przegub 1 front cover v20 (Autodesk Fusion 360 design; units mm, degrees)
Autodesk Fusion 360 part; units mm, degrees
derive "derive" from "Robot asembly v98"
sketch "Sketch1" plane through (0, -130, 0) normal (0, -1, 0) x (1, 0, 0)
  line L0 (-73, -52.5227) -> (-73, -58.5227)
  line L1 (-73, -58.5227) -> (73, -58.5227)
  line L2 (73, -58.5227) -> (73, -52.5227)
  line L3 (73, -52.5227) -> (68, -52.5227)
  line L4 (-68, -54.5227) -> (-68, -52.5227)
  line L5 (-68, -52.5227) -> (-73, -52.5227)
  line L6 (76, -4.5227) -> (73, -4.5227)
  line L7 (73, -4.5227) -> (73, -58.5227)
  line L8 (73, -58.5227) -> (76, -58.5227)
  line L9 (76, -58.5227) -> (76, -4.5227)
  line L10 (73, -4.5227) -> (76, -4.5227)
  arc A0 (76, -4.5227) -> (70, 1.4773) centre (70, -4.5227) ccw
  line L11 (70, 1.4773) -> (70, -1.5227)
  arc A1 (73, -4.5227) -> (70, -1.5227) centre (70, -4.5227) ccw
  line L12 (70, 1.4773) -> (-70, 1.4773)
  line L13 (-70, 1.4773) -> (-70, -1.5227)
  line L14 (-70, -1.5227) -> (70, -1.5227)
  line L15 (70, -1.5227) -> (70, 1.4773)
  line L16 (-76, -4.5227) -> (-73, -4.5227)
  arc A2 (-70, -1.5227) -> (-73, -4.5227) centre (-70, -4.5227) ccw
  line L17 (-70, -1.5227) -> (-70, 1.4773)
  arc A3 (-70, 1.4773) -> (-76, -4.5227) centre (-70, -4.5227) ccw
  line L18 (-73, -4.5227) -> (-76, -4.5227)
  line L19 (-76, -4.5227) -> (-76, -58.5227)
  line L20 (-76, -58.5227) -> (-73, -58.5227)
  line L21 (-73, -58.5227) -> (-73, -4.5227)
  line L22 (69, -5.5227) -> (69, -59.157)
  line L23 (-69, -5.5227) -> (69, -5.5227)
  line L24 (-69, -59.157) -> (-69, -5.5227)
  circle A4 centre (55, -28.5227) radius 12
  line L25 (68.85, -12.1227) -> (41.15, -12.1227) construction
  line L26 (41.15, -12.1227) -> (41.15, -44.9227) construction
  line L27 (41.15, -44.9227) -> (68.85, -44.9227) construction
  line L28 (68.85, -44.9227) -> (68.85, -12.1227) construction
  line L29 (68.85, -12.1227) -> (41.15, -44.9227) construction
  line L30 (41.15, -12.1227) -> (68.85, -44.9227) construction
  circle A5 centre (45.3218, -17.0626) radius 2
  circle A6 centre (64.6782, -39.9828) radius 2
  line L31 (55, -28.5227) -> (68.85, -16.8262) construction
  line L32 (30.15, -12.5227) -> (30.15, -44.5227) construction
  circle A7 centre (30.15, -44.5227) radius 2
  circle A8 centre (30.15, -12.5227) radius 2
  line L33 (24.65, -17.0227) -> (35.65, -17.0227)
  line L34 (24.65, -17.0227) -> (24.65, -40.0227)
  line L35 (24.65, -40.0227) -> (35.65, -40.0227)
  line L36 (35.65, -40.0227) -> (35.65, -17.0227)
  line L37 (30.15, -28.5227) -> (35.65, -28.5227) construction
  line L38 (22.15, -7.5227) -> (38.15, -7.5227) construction
  line L39 (38.15, -7.5227) -> (38.15, -49.5227) construction
  line L40 (38.15, -49.5227) -> (22.15, -49.5227) construction
  line L41 (22.15, -49.5227) -> (22.15, -7.5227) construction
  line L42 (22.15, -7.5227) -> (38.15, -49.5227) construction
  line L43 (38.15, -7.5227) -> (22.15, -49.5227) construction
  line L44 (-73, -58.5227) -> (82.029, -58.5227)
  line L45 (69, -54.5227) -> (-69, -54.5227)
  point P0 (55, -28.5227)
  point P1 (30.15, -28.5227)
  point P2 (30.15, -28.5227)
  dimension "d2" = 24
  dimension "d3" = 27.7
  dimension "d4" = 32.8
  dimension "d5" = 4
  dimension "d6" = 4
  dimension "d7" = 30
  dimension "d9" = 4
  dimension "d10" = 4
  dimension "d11" = 32
  dimension "d12" = 23
  dimension "d13" = 11
  dimension "d14" = 16
  dimension "d15" = 42
  dimension "d49" = 4
  dimension "d52" = 3
  dimension "d53" = 14
  dimension "d54" = 57
  dimension "d55" = 4
  dimension "d56" = 30
  dimension "d57" = 30
  dimension "d58" = 60
  constraint horizontal L25
  constraint perpendicular L25 L26
  constraint parallel L25 L27
  constraint parallel L26 L28
  constraint coincident L29 P0
  constraint coincident L30 P0
  constraint coincident P0 A4.centre
  constraint coincident L30 A5.centre
  constraint coincident L30 A6.centre
  constraint perpendicular L30 L31
  constraint symmetric A5.centre A6.centre L31
  constraint coincident L28 L31.end
  constraint vertical L32
  constraint coincident L32.end A7.centre
  constraint coincident L32.start A8.centre
  constraint horizontal L33
  constraint perpendicular L33 L34
  constraint perpendicular L34 L35
  constraint perpendicular L35 L36
  constraint symmetric L32 L34 L36
  constraint midpoint L32 P2
  constraint midpoint L36 L37.end
  constraint symmetric L33 L35 L37
  constraint coincident P2 P1
  constraint horizontal L38
  constraint perpendicular L38 L39
  constraint parallel L38 L40
  constraint parallel L39 L41
  constraint coincident L42 P2
  constraint coincident L43 P2
  constraint horizontal L44
  constraint perpendicular L23 L24
  constraint coincident L22 L45.start
  constraint coincident L24 L45.end
  constraint perpendicular L24 L45
  constraint coincident L0.end L1.start
  measures "d2" diameter of A4
  measures "d3" distance of L25.start L25.end
  measures "d4" distance of L25.end L26.end
  measures "d5" diameter of A5
  measures "d6" diameter of A6
  measures "d7" distance of A5.centre A6.centre
  measures "d9" diameter of A7
  measures "d10" diameter of A8
  measures "d11" distance of L32.end L32.start
  measures "d12" distance of L35.end L33.end
  measures "d13" distance of L33.start L33.end
  measures "d14" distance of L39.end L40.end
  measures "d15" distance of L38.start L40.end
  measures "d49" distance of L21 L24
  measures "d52" distance of L26 L39
  measures "d53" distance of L22 P0
  measures "d54" distance of L14 L44
  measures "d55" distance of L44 L45
  measures "d56" distance of P2 L44
  measures "d57" distance of P0 L44
  measures "d58" distance of L12 L44
extrude "Extrude1" add sketch "Sketch1" against normal blind 7 contours L0 L1 L5 L21 L24 L44 | L3 L5 L7 A1 L14 A2 L21 L22 L23 L24 | L1 L22 L24 L44 L45 | L1 L2 L3 L7 L22 L44
extrude "Extrude2" add sketch "Sketch1" against normal blind 2 contours L4 L5 L22 L23 L24 L45
extrude "Extrude3" add sketch "Sketch1" along normal blind 2
chamfer "Chamfer1" distance 1 angle 45 5 edges at (-74.2426, -132, -0.2801) (0, -132, 1.4773) (74.2426, -132, -0.2801) (76, -132, -31.5227) (-76, -132, -31.5227)
sketch "Sketch2" plane through (-73, 0, 0) normal (-1, 0, 0) x (0, -1, 0)
  line L0 (130, -58.5227) -> (130, -4.5227)
  line L1 (130, -4.5227) -> (123, -4.5227)
  line L2 (123, -4.5227) -> (123, -58.5227)
  circle A0 centre (126, -48.5227) radius 1.5
  circle A1 centre (126, -14.5227) radius 1.5
  circle A2 centre (126, -14.5227) radius 2
  circle A3 centre (126, -48.5227) radius 2
  line L3 (123, -58.5227) -> (130, -58.5227)
  dimension "d27" = 4
  dimension "d28" = 4
  constraint concentric A1 A2
  constraint concentric A0 A3
  measures "d27" diameter of A2
  measures "d28" diameter of A3
sketch "Sketch3" plane through (0, 0, -1.5227) normal (0, 0, 1) x (-1, 0, 0)
  line L0 (70, 130) -> (-70, 130)
  line L1 (-70, 130) -> (-70, 123)
  line L2 (-70, 123) -> (70, 123)
  line L3 (70, 123) -> (70, 130)
  circle A0 centre (60, 126) radius 1.5
  circle A1 centre (-60, 126) radius 1.5
  circle A2 centre (-20, 126) radius 1.5
  circle A3 centre (20, 126) radius 1.5
  circle A4 centre (60, 126) radius 2
  circle A5 centre (20, 126) radius 2
  circle A6 centre (-20, 126) radius 2
  circle A7 centre (-60, 126) radius 2
  dimension "d29" = 4
  dimension "d30" = 4
  dimension "d31" = 4
  dimension "d32" = 4
  constraint concentric A0 A4
  constraint concentric A3 A5
  constraint concentric A2 A6
  constraint concentric A1 A7
  measures "d29" diameter of A4
  measures "d30" diameter of A5
  measures "d31" diameter of A6
  measures "d32" diameter of A7
sketch "Sketch4" plane through (73, 0, 0) normal (1, 0, 0) x (0, 1, 0)
  line L0 (-130, -4.5227) -> (-130, -58.5227)
  line L1 (-123, -58.5227) -> (-123, -4.5227)
  line L2 (-123, -4.5227) -> (-130, -4.5227)
  circle A0 centre (-126, -48.5227) radius 1.5
  circle A1 centre (-126, -14.5227) radius 1.5
  circle A2 centre (-126, -14.5227) radius 2
  circle A3 centre (-126, -48.5227) radius 2
  line L3 (-130, -58.5227) -> (-123, -58.5227)
  dimension "d33" = 4
  dimension "d34" = 4
  constraint concentric A1 A2
  constraint concentric A0 A3
  measures "d33" diameter of A2
  measures "d34" diameter of A3
sketch "Sketch5" plane through (0, 0, -58.5227) normal (0, 0, -1) x (1, 0, 0)
  line L0 (68, 130) -> (-68, 130)
  line L1 (-68, 130) -> (-68, 123)
  line L2 (-68, 123) -> (68, 123)
  line L3 (68, 123) -> (68, 130)
  circle A0 centre (-60, 126) radius 1.5
  circle A1 centre (-20, 126) radius 1.5
  circle A2 centre (20, 126) radius 1.5
  circle A3 centre (60, 126) radius 1.5
  circle A4 centre (-60, 126) radius 2
  circle A5 centre (-20, 126) radius 2
  circle A6 centre (20, 126) radius 2
  circle A7 centre (60, 126) radius 2
  line L4 (-75, 132) -> (-76, 131)
  line L5 (-76, 131) -> (-76, 130)
  line L6 (-76, 130) -> (-73, 130)
  line L7 (-73, 130) -> (-73, 123)
  line L8 (-73, 123) -> (-69, 123)
  line L9 (73, 123) -> (73, 130)
  line L10 (73, 130) -> (76, 130)
  line L11 (76, 130) -> (76, 131)
  line L12 (76, 131) -> (75, 132)
  line L13 (75, 132) -> (-75, 132)
  line L14 (-69, 123) -> (-69, 130)
  line L15 (-69, 130) -> (69, 130)
  line L16 (69, 130) -> (69, 123)
  line L17 (69, 123) -> (73, 123)
  line L18 (-75, 132) -> (-76, 131)
  line L19 (-76, 131) -> (-76, 130)
  line L20 (-76, 130) -> (-73, 130)
  line L21 (-73, 130) -> (-73, 123)
  line L22 (-73, 123) -> (73, 123)
  line L23 (73, 123) -> (73, 130)
  line L24 (73, 130) -> (76, 130)
  line L25 (76, 130) -> (76, 131)
  line L26 (76, 131) -> (75, 132)
  line L27 (75, 132) -> (-75, 132)
  dimension "d35" = 4
  dimension "d36" = 4
  dimension "d37" = 4
  dimension "d38" = 4
  constraint concentric A0 A4
  constraint concentric A1 A5
  constraint concentric A2 A6
  constraint concentric A3 A7
  measures "d35" diameter of A4
  measures "d36" diameter of A5
  measures "d37" diameter of A6
  measures "d38" diameter of A7
extrude "Extrude4" cut sketch "Sketch4" against normal blind 4 contours A0 | A1 | A2 | A3
extrude "Extrude5" cut sketch "Sketch3" against normal blind 4 contours A0 | A1 | A2 | A3 | A4 | A5 | A6 | A7
extrude "Extrude6" cut sketch "Sketch2" against normal blind 4 contours A0 | A1 | A2 | A3
extrude "Extrude7" cut sketch "Sketch5" against normal blind 4 contours A0 | A1 | A2 | A3 | A4 | A5 | A6 | A7
sketch "Sketch6" plane through (0, -132, 0) normal (0, -1, 0) x (1, 0, 0)
  line L0 (-75, -4.5227) -> (-75, -58.5227)
  line L1 (-75, -58.5227) -> (75, -58.5227)
  line L2 (75, -58.5227) -> (75, -4.5227)
  arc A0 (75, -4.5227) -> (70, 0.4773) centre (70, -4.5227) ccw
  line L3 (70, 0.4773) -> (-70, 0.4773)
  arc A1 (-70, 0.4773) -> (-75, -4.5227) centre (-70, -4.5227) ccw
  circle A2 centre (55, -28.5227) radius 12
  circle A3 centre (30.15, -44.5227) radius 2
  circle A4 centre (30.15, -12.5227) radius 2
  line L4 (24.65, -40.0227) -> (24.65, -17.0227)
  line L5 (24.65, -17.0227) -> (35.65, -17.0227)
  line L6 (35.65, -17.0227) -> (35.65, -40.0227)
  line L7 (35.65, -40.0227) -> (24.65, -40.0227)
  circle A5 centre (64.6782, -39.9828) radius 2
  circle A6 centre (45.3218, -17.0626) radius 2
  line L8 (69, -54.5227) -> (69, -5.5227)
  line L9 (69, -5.5227) -> (-69, -5.5227)
  line L10 (-69, -5.5227) -> (-69, -54.5227)
  line L11 (-69, -54.5227) -> (69, -54.5227)
  line L12 (-73, -58.5227) -> (-73, -4.5227)
  arc A7 (-70, -1.5227) -> (-73, -4.5227) centre (-70, -4.5227) ccw
  line L13 (-70, -1.5227) -> (70, -1.5227)
  arc A8 (73, -4.5227) -> (70, -1.5227) centre (70, -4.5227) ccw
  line L14 (73, -4.5227) -> (73, -58.5227)
  line L15 (73, -58.5227) -> (-73, -58.5227)
  line L16 (0, -1.5227) -> (0, -54.5227) construction
  line L17 (-62.5, -8.5227) -> (-66, -14.5849)
  line L18 (-66, -14.5849) -> (-59, -14.5849)
  line L19 (-59, -14.5849) -> (-62.5, -8.5227)
  line L20 (-62.5, -8.5227) -> (-61.1144, -8.5227) construction
  line L21 (-59, -15.7849) -> (-66, -15.7849)
  line L22 (-66, -15.7849) -> (-62.5, -21.8471)
  line L23 (-62.5, -21.8471) -> (-59, -15.7849)
  line L24 (-62.5, -23.0471) -> (-66, -29.1092)
  line L25 (-66, -29.1092) -> (-59, -29.1092)
  line L26 (-59, -29.1092) -> (-62.5, -23.0471)
  line L27 (-59, -30.3092) -> (-66, -30.3092)
  line L28 (-66, -30.3092) -> (-62.5, -36.3714)
  line L29 (-62.5, -36.3714) -> (-59, -30.3092)
  line L30 (-62.5, -37.5714) -> (-66, -43.6336)
  line L31 (-66, -43.6336) -> (-59, -43.6336)
  line L32 (-59, -43.6336) -> (-62.5, -37.5714)
  line L33 (-59, -44.8336) -> (-66, -44.8336)
  line L34 (-66, -44.8336) -> (-62.5, -50.8958)
  line L35 (-62.5, -50.8958) -> (-59, -44.8336)
  line L36 (-62.5, -8.5227) -> (-62.5, -50.8958) construction
  line L37 (-61.1144, -8.5227) -> (-57.6144, -14.5849)
  line L38 (-57.6144, -14.5849) -> (-54.1144, -8.5227)
  line L39 (-54.1144, -8.5227) -> (-61.1144, -8.5227)
  line L40 (-54.1144, -21.8471) -> (-57.6144, -15.7849)
  line L41 (-61.1144, -21.8471) -> (-54.1144, -21.8471)
  line L42 (-57.6144, -15.7849) -> (-61.1144, -21.8471)
  line L43 (-54.1144, -50.8958) -> (-57.6144, -44.8336)
  line L44 (-57.6144, -44.8336) -> (-61.1144, -50.8958)
  line L45 (-61.1144, -50.8958) -> (-54.1144, -50.8958)
  line L46 (-54.1144, -36.3714) -> (-57.6144, -30.3092)
  line L47 (-57.6144, -30.3092) -> (-61.1144, -36.3714)
  line L48 (-61.1144, -36.3714) -> (-54.1144, -36.3714)
  line L49 (-57.6144, -29.1092) -> (-54.1144, -23.0471)
  line L50 (-54.1144, -23.0471) -> (-61.1144, -23.0471)
  line L51 (-61.1144, -23.0471) -> (-57.6144, -29.1092)
  line L52 (-57.6144, -43.6336) -> (-54.1144, -37.5714)
  line L53 (-54.1144, -37.5714) -> (-61.1144, -37.5714)
  line L54 (-61.1144, -37.5714) -> (-57.6144, -43.6336)
  line L55 (-62.5, -21.8471) -> (-61.1144, -21.8471) construction
  line L56 (-62.5, -23.0471) -> (-61.1144, -23.0471) construction
  line L57 (-62.5, -36.3714) -> (-61.1144, -36.3714) construction
  line L58 (-62.5, -37.5714) -> (-61.1144, -37.5714) construction
  line L59 (-62.5, -50.8958) -> (-61.1144, -50.8958) construction
  point P0 (-62.5, -30.3092)
  point P1 (-62.5, -43.6336)
  point P2 (-62.5, -44.8336)
  point P3 (-62.5, -15.7849)
  dimension "d68" = 60
  dimension "d69" = 60
  dimension "d70" = 7
  dimension "d71" = 3
  dimension "d72" = 3
  dimension "d83" = 60
  dimension "d84" = 60
  dimension "d85" = 7
  dimension "d86" = 60
  dimension "d87" = 60
  dimension "d88" = 7
  dimension "d89" = 60
  dimension "d90" = 60
  dimension "d91" = 7
  dimension "d92" = 60
  dimension "d93" = 60
  dimension "d94" = 7
  dimension "d95" = 60
  dimension "d96" = 60
  dimension "d97" = 7
  dimension "d98" = 1.2
  dimension "d99" = 1.2
  dimension "d100" = 1.2
  dimension "d101" = 1.2
  dimension "d102" = 1.2
  dimension "d103" = 60
  dimension "d104" = 60
  dimension "d105" = 7
  dimension "d106" = 60
  dimension "d107" = 60
  dimension "d108" = 7
  dimension "d110" = 1.2
  dimension "d111" = 60
  dimension "d112" = 60
  dimension "d113" = 7
  dimension "d114" = 60
  dimension "d115" = 60
  dimension "d116" = 7
  dimension "d117" = 60
  dimension "d118" = 60
  dimension "d119" = 7
  dimension "d120" = 60
  dimension "d121" = 60
  dimension "d122" = 7
  dimension "d123" = 1.2
  dimension "d124" = 1.2
  dimension "d125" = 1.2
  dimension "d126" = 1.2
  dimension "d127" = 1.2
  constraint midpoint L13 L16.start
  constraint midpoint L11 L16.end
  constraint horizontal L18
  constraint horizontal L25
  constraint horizontal L31
  constraint perpendicular L33 L36
  constraint midpoint L27 P0
  constraint midpoint L31 P1
  constraint midpoint L33 P2
  constraint coincident L36 P1
  constraint coincident L28.end L36
  constraint coincident L24.start L36
  constraint midpoint L21 P3
  constraint coincident L36 P3
  constraint coincident L20.end L37.start
  constraint horizontal L20
  constraint perpendicular L36 L55
  constraint coincident L41.start L42.end
  constraint perpendicular L36 L56
  constraint perpendicular L36 L57
  constraint perpendicular L36 L58
  constraint perpendicular L36 L59
  constraint coincident L44.end L45.start
  constraint coincident L53.end L54.start
  constraint coincident L47.end L48.start
  constraint coincident L50.end L51.start
  measures "d68" angle of L17 L18
  measures "d69" angle of L17 L19
  measures "d70" distance of L17.start L18.end
  measures "d71" distance of L10 L17.end
  measures "d72" distance of L9 L17.start
  measures "d83" angle of L21 L22
  measures "d84" angle of L21 L23
  measures "d85" distance of L22.end L21.start
  measures "d86" angle of L24 L25
  measures "d87" angle of L24 L26
  measures "d88" distance of L25.end L24.start
  measures "d89" angle of L27 L28
  measures "d90" angle of L27 L29
  measures "d91" distance of L28.end L27.start
  measures "d92" angle of L30 L31
  measures "d93" angle of L30 L32
  measures "d94" distance of L31.end L30.start
  measures "d95" angle of L33 L34
  measures "d96" angle of L33 L35
  measures "d97" distance of L34.end L33.start
  measures "d98" distance of L18 L21
  measures "d99" vertical distance of L22.end L24.start
  measures "d100" distance of L25 L27
  measures "d101" vertical distance of L28.end L30.start
  measures "d102" distance of L31 L33
  measures "d103" angle of L37 L38
  measures "d104" angle of L37 L39
  measures "d105" distance of L38.end L20.end
  measures "d106" angle of L40 L42
  measures "d107" angle of L40 L41
  measures "d108" distance of L41.start L40.start
  measures "d110" distance of L19 L37
  measures "d111" angle of L43 L44
  measures "d112" angle of L43 L45
  measures "d113" distance of L44.end L43.start
  measures "d114" angle of L46 L47
  measures "d115" angle of L46 L48
  measures "d116" distance of L47.end L46.start
  measures "d117" angle of L49 L51
  measures "d118" angle of L50 L51
  measures "d119" distance of L49.end L50.end
  measures "d120" angle of L52 L54
  measures "d121" angle of L53 L54
  measures "d122" distance of L52.end L53.end
  measures "d123" distance of L23 L42
  measures "d124" distance of L26 L51
  measures "d125" distance of L29 L47
  measures "d126" distance of L32 L54
  measures "d127" distance of L35 L44
extrude "Extrude8" cut sketch "Sketch6" against normal blind 4 contours L17 L18 L19 | L21 L22 L23 | L24 L25 L26 | L27 L28 L29 | L30 L31 L32 | L33 L34 L35 | L37 L38 L39 | L40 L41 L42 | L43 L44 L45 | L46 L47 L48 | L49 L50 L51 | L52 L53 L54
pattern_linear "R-Pattern2" count 8 spacing 9.77 along (1, 0, 0) of "Extrude8"
equation "d9 = d10"
equation "d28 = d27"
equation "d29 = d32"
equation "d30 = d32"
equation "d31 = d32"
equation "d34 = d33"
equation "d56 = d58 / 2"
equation "d57 = d56"
equation "d82 = 1.2 mm"
equation "d98 = d82"
equation "d99 = d82"
equation "d100 = d82"
equation "d101 = d82"
equation "d102 = d82"
equation "d110 = d98"
equation "d123 = d98"
equation "d124 = d98"
equation "d125 = d98"
equation "d126 = d98"
equation "d127 = d98"
